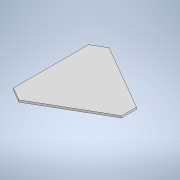
# Autodesk Inventor part: PCB_Top
Saved by Autodesk Inventor 2020.2 (Build 242310000, 310)
## iProperties
Created: 2021-02-25
Part Number: PCB_Top
Material: Generic
Document SubType Name: Modeling
Designer: saika
Density: 1 g/cm^3
Appearance: Default
Author: saika
Autodesk Inventor part; units mm, degrees
ref_plane "YZ Plane" through (0, 0, 0) normal (1, 0, 0) x (0, 1, 0)
ref_plane "XZ Plane" through (0, 0, 0) normal (0, 1, 0) x (-1, 0, 0)
ref_plane "XY Plane" through (0, 0, 0) normal (0, 0, 1) x (1, 0, 0)
sketch "Sketch2" plane through (0, 0, 0) normal (0, 1, 0) x (-1, 0, 0)
  line L0 (-38.1051, 6) -> (13.8564, 36)
  line L1 (-38.1051, 6) -> (-38.1051, -6)
  line L2 (13.8564, -36) -> (-38.1051, -6)
  line L3 (13.8564, -36) -> (24.2487, -30)
  line L4 (24.2487, -30) -> (24.2487, 30)
  line L5 (13.8564, 36) -> (24.2487, 30)
  point P0 (0, 0)
  point P1 (0, 0)
  constraints: 12 end point
extrude "Extrusion1" add sketch "Sketch2" along normal blind 1.6
body "Solid1"
